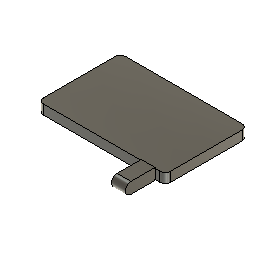
3M 6000 Series Electronic Box v30 (Autodesk Fusion 360 archive; units mm, degrees)
design "Power Bank"
Autodesk Fusion 360 part; units mm, degrees
sketch "Sketch1" plane through (0, 0, 0) normal (0, 0, 1) x (1, 0, 0)
  line L0 (48.15, 31.15) -> (-48.15, 31.15)
  line L1 (-48.15, 31.15) -> (-48.15, -31.15)
  line L2 (-48.15, -31.15) -> (48.15, -31.15)
  line L3 (48.15, -31.15) -> (48.15, 31.15)
  line L4 (48.15, 31.15) -> (-48.15, -31.15) construction
  line L5 (-48.15, 31.15) -> (48.15, -31.15) construction
  line L6 (0, 0) -> (48.15, 0) construction
  circle A0 centre (40.15, 0) radius 1.5
  dimension "d1" = 96.3
  dimension "d2" = 62.3
  dimension "d10" = 3
  dimension "d11" = 8
  constraint horizontal L0
  constraint perpendicular L0 L1
  constraint parallel L0 L2
  constraint parallel L1 L3
  constraint coincident L4 L6.start
  constraint coincident L5 L6.start
  constraint coincident L6.start origin
  constraint midpoint L3 L6.end
  constraint coincident L6 A0.centre
  measures "d1" distance of L1.end L2.end
  measures "d2" distance of L0.end L1.end
  measures "d10" diameter of A0
  measures "d11" distance of L3 A0.centre
extrude "Extrude1" add sketch "Sketch1" along normal blind 7.3 contours L0 L1 L2 L3 | A0
fillet "Fillet1" radius 4 4 edges at (-48.15, -31.15, 3.65) (48.15, -31.15, 3.65) (48.15, 31.15, 3.65) (-48.15, 31.15, 3.65)
extrude "Extrude2" add sketch "Sketch1" against normal blind 0.2 contours A0
sketch "Sketch3" plane through (0, -31.15, 0) normal (0, -1, 0) x (1, 0, 0)
  line L0 (44.15, 0) -> (44.15, 7.3)
  line L1 (44.15, 7.3) -> (-44.15, 7.3)
  line L2 (-44.15, 7.3) -> (-44.15, 0)
  line L3 (-44.15, 0) -> (44.15, 0)
  line L4 (48.15, 0) -> (48.15, 7.3) construction
  line L5 (48.15, 3.65) -> (35.15, 3.65) construction
  line L6 (40.4, -0.6) -> (29.9, -0.6)
  line L7 (29.9, -0.6) -> (29.9, 7.9)
  line L8 (29.9, 7.9) -> (40.4, 7.9)
  line L9 (40.4, 7.9) -> (40.4, -0.6)
  line L10 (40.4, -0.6) -> (29.9, 7.9) construction
  line L11 (29.9, -0.6) -> (40.4, 7.9) construction
  point P0 (35.15, 3.65)
  dimension "d16" = 13
  dimension "d17" = 10.5
  dimension "d18" = 8.5
  constraint midpoint L4 L5.start
  constraint perpendicular L0 L5
  constraint horizontal L6
  constraint perpendicular L6 L7
  constraint parallel L6 L8
  constraint parallel L7 L9
  constraint coincident L10 P0
  constraint coincident L11 P0
  constraint coincident P0 L5.end
  measures "d16" distance of L5.start P0
  measures "d17" distance of L7.end L8.end
  measures "d18" distance of L6.end L7.end
extrude "Extrude3" add sketch "Sketch3" along normal blind 22.5 contours L3 L6 L7 L9 | L1 L3 L7 L9 | L1 L7 L8 L9
fillet "Fillet2" radius 4.25 2 edges at (35.15, -53.65, -0.6) (35.15, -53.65, 7.9)
equation "d1 = powerBankLength"
equation "d2 = powerBankWidth"
equation "clearanceStationary = 0.125 mm"
equation "clearanceMoving = 2 * clearanceStationary"
equation "powerBankWidth = 62.3 mm"
equation "powerBankLength = 96.3 mm"
equation "powerBankHeight = 7.3 mm"
equation "d8 = powerBankHeight"
equation "d17 = usbPlugWidth"
equation "d18 = usbPlugHeight"
equation "usbPlugWidth = 10.5 mm"
equation "usbPlugHeight = 8.5 mm"
equation "usbPlugLength = 22.5 mm"
equation "d22 = usbPlugLength"
equation "d25 = usbPlugHeight / 2"
